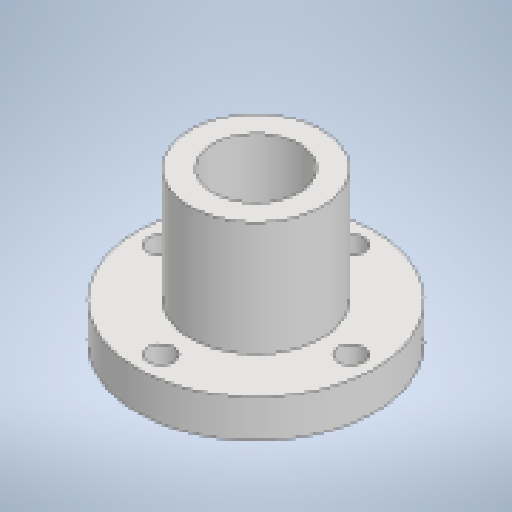
# Autodesk Inventor part: 18mm hub
Saved by Autodesk Inventor 2025 (Build 290162000, 162)
## iProperties
Created: 2025-09-09
Part Number: 18mm hub
Material: 一般
Document SubType Name: Modeling
Designer: gavin
Density: 1 g/cm^3
Appearance: 預設
Author: gavin
Autodesk Inventor part; units mm, degrees
ref_plane "YZ Plane" through (0, 0, 0) normal (1, 0, 0) x (0, 1, 0)
ref_plane "XZ Plane" through (0, 0, 0) normal (0, 1, 0) x (-1, 0, 0)
ref_plane "XY Plane" through (0, 0, 0) normal (0, 0, 1) x (1, 0, 0)
sketch "草圖1" plane through (0, 0, 0) normal (0, 1, 0) x (-1, 0, 0)
  circle A0 centre (0, 0) radius 25
  circle A1 centre (0, 0) radius 20 construction
  circle A2 centre (20, 0) radius 2.75
  circle A3 centre (0, 20) radius 2.75
  circle A4 centre (-20, 0) radius 2.75
  circle A5 centre (0, -20) radius 2.75
  circle A6 centre (0, 0) radius 9
  dimension "d1" = 40
  dimension "d0" = 50
  dimension "d2" = 5.5
  dimension "d5" = 360
  dimension "d7" = 18
  constraints: 6 centre point, 3 coincident, 1 horizontal alignment, 11 other
  measures "d0" diameter of A0
  measures "d2" diameter of A2
  measures "d7" diameter of A6
extrude "擠出1" add sketch "草圖1" along normal blind 8
sketch "草圖2" plane through (0, 8, 0) normal (0, 1, 0) x (1, 0, 0)
  circle A0 centre (0, 0) radius 9 projected
  circle A1 centre (0, 0) radius 13.93
  dimension "d10" = 27.86
  constraints: 1 centre point, 1 coincident
  measures "d10" diameter of A1
extrude "擠出2" add sketch "草圖2" along normal blind 24
